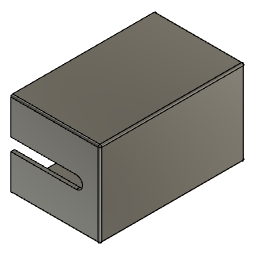
BlindMotorBox v1 (Autodesk Fusion 360 design; units mm, degrees)
Autodesk Fusion 360 part; units mm, degrees
sketch "Sketch1" plane through (0, 0, 0) normal (1, 0, 0) x (0, 1, 0) in component "Box"
  line L0 (0, 0) -> (80, 0)
  line L1 (80, 0) -> (80, 47)
  line L2 (80, 47) -> (0, 47)
  line L3 (0, 47) -> (0, 0)
  dimension "d1" = 80
  dimension "d2" = 47
  constraint horizontal L0
  constraint vertical L1
  constraint horizontal L2
  constraint vertical L3
  constraint coincident L0.start L3.end
  measures "d1" distance of L0.start L0.end
  measures "d2" distance of L0.start L2.end
extrude "Extrude1" add sketch "Sketch1" along normal blind 49 in component "Box"
sketch "Sketch2" plane through (0, 0, 0) normal (-1, 0, 0) x (0, -1, 0) in component "Box"
  line L0 (0, 0) -> (0, 47)
  line L1 (0, 47) -> (-80, 47)
  line L2 (-80, 47) -> (-80, 0)
  line L3 (-80, 0) -> (0, 0)
  line L4 (-78, 2) -> (-2, 2)
  line L5 (-2, 2) -> (-2, 45)
  line L6 (-2, 45) -> (-78, 45)
  line L7 (-78, 45) -> (-78, 2)
  dimension "d5" = -2
extrude "Extrude2" cut sketch "Sketch2" against normal blind 47 contours L4 L5 L6 L7 in component "Box"
sketch "Sketch3" plane through (0, 0, 0) normal (0, 1, 0) x (1, 0, 0) in component "Box"
  circle A0 centre (36, -23.5) radius 3.5
  line L0 (0, -47) -> (0, 0)
  line L1 (0, 0) -> (49, 0)
  line L2 (36, -20) -> (0, -20)
  line L3 (36, -27) -> (0, -27)
  dimension "d8" = 7
  dimension "d12" = 36
  dimension "d13" = 23.5
  constraint coincident A0 L2.start
  constraint coincident L0 L2.end
  constraint tangent A0 L2
  constraint perpendicular L0 L2
  constraint coincident A0 L3.start
  constraint coincident L0 L3.end
  constraint tangent A0 L3
  constraint perpendicular L0 L3
  measures "d8" diameter of A0
  measures "d12" distance of A0.centre L0
  measures "d13" distance of A0.centre L1
extrude "Extrude3" cut sketch "Sketch3" along normal up to surface (2 mm away) in component "Box"
fillet "Fillet1" radius 1 8 edges at (24.5, 0, 47) (24.5, 80, 47) (24.5, 80, 0) (24.5, 0, 0) (49, 40, 47) (49, 40, 0) (49, 0, 23.5) (49, 80, 23.5) in component "Box"
component "Box" placed x (1, 0, 0) y (0, 1, 0) z (0, 0, 1) at (0, 0, 0)
